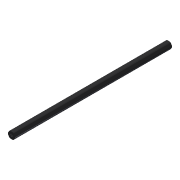
# Autodesk Inventor part: ThunderHex
Saved by Autodesk Inventor 2015 (Build 190159000, 159)
## iProperties
Created: 2014-12-18
Part Number: ThunderHex
Material: Aluminum 6061
Document SubType Name: Modeling
Designer: Nemo
Density: 2.7 g/cm^3
Appearance: Rubber - Black
Author: Nemo
Autodesk Inventor part; units mm, degrees
ref_plane "YZ Plane" through (0, 0, 0) normal (1, 0, 0) x (0, 1, 0)
ref_plane "XZ Plane" through (0, 0, 0) normal (0, 1, 0) x (-1, 0, 0)
ref_plane "XY Plane" through (0, 0, 0) normal (0, 0, 1) x (1, 0, 0)
sketch "ThunderHex" plane through (0, 0, 0) normal (0, 0, 1) x (1, 0, 0)
  line L0 (0, 0) -> (5.1191, 0)
  line L1 (6.801, -0.9711) -> (9.3605, -5.4043)
  arc A0 (0, 0) -> (-1.682, -0.9711) centre (2.5595, -6.3754) ccw
  arc A1 (9.3605, -7.3465) -> (9.3605, -5.4043) centre (2.5595, -6.3754) ccw
  circle A2 centre (2.5595, -6.3754) radius 2.55
  line L2 (-4.2415, -5.4043) -> (-1.682, -0.9711)
  arc A3 (-4.2415, -5.4043) -> (-4.2415, -7.3465) centre (2.5595, -6.3754) ccw
  line L3 (-1.682, -11.7797) -> (-4.2415, -7.3465)
  arc A4 (-1.682, -11.7797) -> (0, -12.7508) centre (2.5595, -6.3754) ccw
  line L4 (5.1191, -12.7508) -> (0, -12.7508)
  arc A5 (5.1191, -12.7508) -> (6.801, -11.7797) centre (2.5595, -6.3754) ccw
  line L5 (9.3605, -7.3465) -> (6.801, -11.7797)
  arc A6 (6.801, -0.9711) -> (5.1191, 0) centre (2.5595, -6.3754) ccw
  point P0 (2.5595, -6.3754)
sketch "Sketch1" plane through (0, 0, 0) normal (0, 0, 1) x (1, 0, 0)
  line L0 (-2.5595, 6.3754) -> (2.5595, 6.3754)
  line L1 (4.2415, 5.4043) -> (6.801, 0.9711)
  arc A0 (-2.5595, 6.3754) -> (-4.2415, 5.4043) centre (0, 0) ccw
  arc A1 (6.801, -0.9711) -> (6.801, 0.9711) centre (0, 0) ccw
  circle A2 centre (0, 0) radius 2.55
  line L2 (-6.801, 0.9711) -> (-4.2415, 5.4043)
  arc A3 (-6.801, 0.9711) -> (-6.801, -0.9711) centre (0, 0) ccw
  line L3 (-4.2415, -5.4043) -> (-6.801, -0.9711)
  arc A4 (-4.2415, -5.4043) -> (-2.5595, -6.3754) centre (0, 0) ccw
  line L4 (2.5595, -6.3754) -> (-2.5595, -6.3754)
  arc A5 (2.5595, -6.3754) -> (4.2415, -5.4043) centre (0, 0) ccw
  line L5 (6.801, -0.9711) -> (4.2415, -5.4043)
  arc A6 (4.2415, 5.4043) -> (2.5595, 6.3754) centre (0, 0) ccw
  constraints: 1 other
extrude "Extrusion1" add sketch "Sketch1" along normal mid plane 304.8
body "Solid1"
